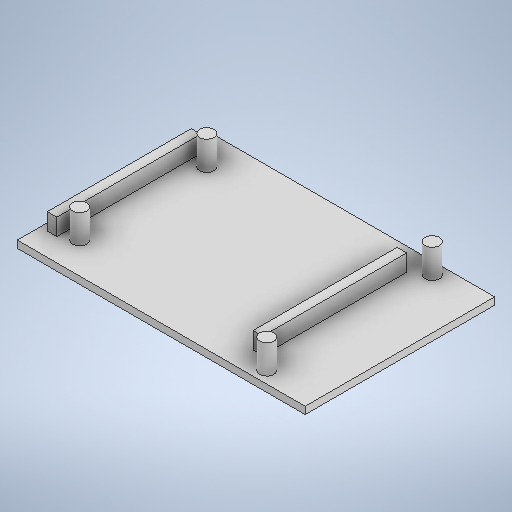
# Autodesk Inventor part: RFID-RC522 Holder 3.1
Saved by Autodesk Inventor 2025.2 (Build 292293000, 293)
## iProperties
Created: 2024-11-16
Part Number: RFID-RC522 Holder 3.1
Material: Generic
Document SubType Name: Modeling
Designer: jurre
Density: 1 g/cm^3
Appearance: Default
Author: jurre
Autodesk Inventor part; units mm, degrees
ref_plane "YZ Plane" through (0, 0, 0) normal (1, 0, 0) x (0, 1, 0)
ref_plane "XZ Plane" through (0, 0, 0) normal (0, 1, 0) x (-1, 0, 0)
ref_plane "XY Plane" through (0, 0, 0) normal (0, 0, 1) x (1, 0, 0)
sketch "Sketch5" plane through (0, 0, 0) normal (0, 1, 0) x (-1, 0, 0)
  line L0 (9.4203, 11.6048) -> (-50.5797, 11.6048)
  line L1 (-50.5797, 11.6048) -> (-50.5797, -27.8952)
  line L2 (-50.5797, -27.8952) -> (9.4203, -27.8952)
  line L3 (9.4203, -27.8952) -> (9.4203, 11.6048)
  line L4 (-36.9794, -23.1452) -> (-34.9794, -23.1452)
  line L5 (-34.9794, -23.1452) -> (-34.9794, 6.8548)
  line L6 (-34.9794, 6.8548) -> (-36.9794, 6.8548)
  line L7 (-36.9794, 6.8548) -> (-36.9794, -23.1452)
  line L8 (7.9203, 6.8548) -> (5.9203, 6.8548)
  line L9 (5.9203, 6.8548) -> (5.9203, -23.1452)
  line L10 (5.9203, -23.1452) -> (7.9203, -23.1452)
  line L11 (7.9203, -23.1452) -> (7.9203, 6.8548)
  circle A0 centre (2.9203, -21.3952) radius 1.5
  circle A1 centre (2.9203, 5.1048) radius 1.5
  circle A2 centre (-40.0797, -25.3952) radius 1.5
  circle A3 centre (-40.0797, 9.1048) radius 1.5
  point P0 (0, 0)
  dimension "d9" = 60
  dimension "d10" = 39.5
  dimension "d24" = 2
  dimension "d25" = 2
  dimension "d26" = 30
  dimension "d27" = 4.75
  dimension "d28" = 4.75
  dimension "d29" = 2
  dimension "d30" = 30
  dimension "d31" = 1.5
  dimension "d32" = 4.75
  dimension "d33" = 4.75
  dimension "d40" = 3
  dimension "d41" = 6.5
  dimension "d42" = 6.5
  dimension "d43" = 3
  dimension "d44" = 6.5
  dimension "d45" = 6.5
  dimension "d46" = 3
  dimension "d47" = 2.5
  dimension "d48" = 10.5
  dimension "d49" = 3
  dimension "d50" = 2.5
  dimension "d51" = 10.5
  constraints: 24 end point, 6 parallel, 4 centre point, 3 horizontal, 3 perpendicular
  measures "d9" distance of L2.end L1.end
  measures "d10" distance of L1.end L0.end
  measures "d24" distance of L6.end L5.end
  measures "d25" distance of L4.start L4.end
  measures "d26" distance of L4.end L5.end
  measures "d27" distance between parallel lines of L0 L6
  measures "d28" distance between parallel lines of L2 L4
  measures "d29" distance of L10.end L9.end
  measures "d30" distance of L9.end L8.end
  measures "d31" distance between parallel lines of L3 L11
  measures "d32" distance between parallel lines of L0 L8
  measures "d33" distance between parallel lines of L2 L10
  measures "d40" diameter of A0
  measures "d41" distance from line of L2 A0.centre
  measures "d42" distance from line of L3 A0.centre
  measures "d43" diameter of A1
  measures "d44" distance from line of L0 A1.centre
  measures "d45" distance from line of L3 A1.centre
  measures "d46" diameter of A2
  measures "d47" distance from line of L2 A2.centre
  measures "d48" distance from line of L1 A2.centre
  measures "d49" diameter of A3
  measures "d50" distance from line of L0 A3.centre
  measures "d51" distance from line of L1 A3.centre
extrude "Extrusion5" add sketch "Sketch5" against normal blind 1.5 contours L3 L2 L1 L0 | L7 L6 L5 L4 | L11 L10 L9 L8 | A0 | A1 | A2 | A3
extrude "Extrusion6" add sketch "Sketch5" along normal blind 6 contours A0 | A1 | A2 | A3
extrude "Extrusion7" add sketch "Sketch5" along normal blind 3.5 contours L7 L6 L5 L4 | L11 L10 L9 L8
body "Solid3"
